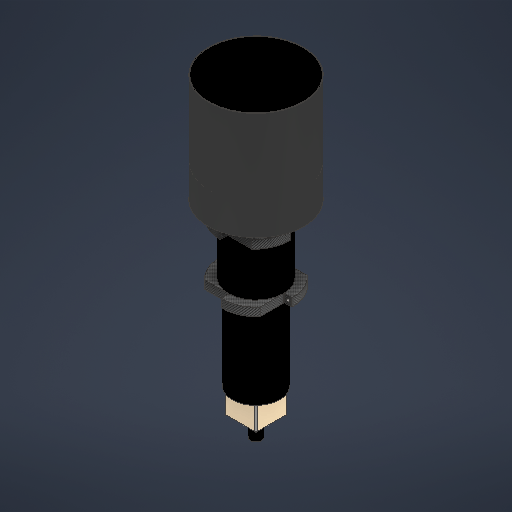
# Autodesk Inventor part: Carbon_Fibre
Saved by Autodesk Inventor 2026.2 (Build 302298000, 298)
## iProperties
Created: 2025-12-09
Part Number: Carbon_Fibre
Material: Steel
Document SubType Name: Modeling
Designer: Thoma
Density: 7.85 g/cm^3
Appearance: Semi-Polished
Mass: 18868.6 g
Surface Area: 2628.33 cm^2
Volume: 2403.64 cm^3
Author: Thoma
Autodesk Inventor part; units mm, degrees
ref_plane "YZ Plane" through (0, 0, 0) normal (1, 0, 0) x (0, 1, 0)
ref_plane "XZ Plane" through (0, 0, 0) normal (0, 1, 0) x (-1, 0, 0)
ref_plane "XY Plane" through (0, 0, 0) normal (0, 0, 1) x (1, 0, 0)
sketch "Sketch1" plane through (0, 0, 0) normal (0, 1, 0) x (-1, 0, 0)
  circle A0 centre (0, 0) radius 43.5
  dimension "d0" = 87
  constraints: 1 centre point, 1 coincident
  measures "d0" diameter of A0
extrude "Extrusion1" add sketch "Sketch1" along normal blind 13
sketch "Sketch2" plane through (0, 13, 0) normal (0, 1, 0) x (1, 0, 0)
  circle A0 centre (0, 0) radius 43.5 projected
  line L0 (0, 55.4914) -> (0, 55.5)
  circle A1 centre (0, 0) radius 43.5 projected
  line L1 (43.5, 0) -> (43.5, 37)
  line L2 (0, 55.5) -> (1, 55.5)
  line L3 (1, 55.5) -> (1, 43.5)
  line L4 (0, 55.4914) -> (0, 55.5)
  arc A2 (43.5, 37) -> (1, 55.5) centre (1, -2.5676) ccw
  line L5 (1, 43.4885) -> (1, 43.5)
  line L6 (-55.5, 1) -> (-43.5, 1)
  arc A3 (-37, 43.5) -> (-55.5, 1) centre (2.5676, 1) ccw
  line L7 (0, 43.5) -> (-37, 43.5)
  line L8 (-1, -55.5) -> (-1, -43.5)
  arc A4 (-43.5, -37) -> (-1, -55.5) centre (-1, 2.5676) ccw
  line L9 (-43.5, 0) -> (-43.5, -37)
  line L10 (55.5, -1) -> (43.5, -1)
  arc A5 (37, -43.5) -> (55.5, -1) centre (-2.5676, -1) ccw
  line L11 (0, -43.5) -> (37, -43.5)
  point P0 (0, 43.5)
  point P1 (43.5, 0)
  point P2 (-55.4914, 0)
  point P3 (0, -55.4914)
  point P4 (55.4914, 0)
  dimension "d3" = 12
  dimension "d75" = 1
  dimension "d91" = 37
  dimension "d92" = 58.0676
  dimension "d93" = 42.5
  dimension "d94" = 0
  dimension "d95" = 87.5
  dimension "d110" = 360
  constraints: 24 end point, 13 point on circle, 4 centre point, 4 vertical, 1 horizontal, 1 parallel, 1 perpendicular, 1 tangent, 39 other
  measures "d3" distance of A1.start L0.end
  measures "d75" distance of L0.end L2.end
  measures "d91" distance of L1.start L1.end
  measures "d92" radius of A2
  measures "d93" distance between parallel lines of L3 L1
  measures "d94" distance from line of point (43.5, 0) L1
extrude "Extrusion2" add sketch "Sketch2" against normal blind 13 contours A0 L5 L3 A2 L1
sketch "Sketch6" plane through (0, 0, 0) normal (0, -1, 0) x (1, 0, 0)
  circle A0 centre (0, 0) radius 43.5
  point P0 (0, 43.5)
  constraints: 1 coincident, 1 vertical alignment, 2 other
sketch "Sketch17" plane through (0, 13, 0) normal (0, 1, 0) x (1, 0, 0)
  circle A0 centre (0, 0) radius 25
  dimension "d141" = 50
  constraints: 1 centre point, 1 coincident
  measures "d141" diameter of A0
extrude "Extrusion16" add sketch "Sketch17" along normal blind 2
sketch "Sketch7" plane through (0, 13, 0) normal (0, 1, 0) x (1, 0, 0)
  circle A0 centre (0, 0) radius 37.5
  dimension "d23" = 75
  constraints: 1 centre point, 1 coincident
  measures "d23" diameter of A0
extrude "Extrusion5" add sketch "Sketch7" along normal blind 15
extrude "Extrusion6" add sketch "Sketch6" along normal blind 79
sketch "Sketch8" plane through (0, -79, 0) normal (0, -1, 0) x (1, 0, 0)
  line L0 (0, -43.5) -> (0, -55.5) projected
  line L1 (0, -43.4937) -> (0, -55.5)
  line L2 (43.4937, 0) -> (55.5, 0)
  line L3 (0, 43.4937) -> (0, 55.5)
  line L4 (-43.4937, 0) -> (-55.5, 0)
  line L5 (-55.5, -2) -> (-43.5, -2)
  circle A0 centre (0, 0) radius 43.5
  line L6 (-43.5, 0) -> (-55.5, 0) projected
  line L7 (-55.5, 0) -> (-55.5, -2)
  line L8 (-43.5, 0) -> (-43.5, -37)
  circle A1 centre (0, 0) radius 43.5 projected
  line L9 (-55.5, 0) -> (-55.5, 1)
  line L10 (-55.5, 1) -> (-43.4885, 1)
  line L11 (0, -43.5) -> (37, -43.5)
  line L12 (-1, -55.5) -> (-1, -43.4885)
  line L13 (2, -55.5) -> (2, -43.5)
  line L14 (0, -55.5) -> (2, -55.5)
  line L15 (0, -55.5) -> (-1, -55.5)
  circle A2 centre (0, 0) radius 43.5
  line L16 (43.5, 0) -> (43.5, 37)
  line L17 (55.5, -1) -> (43.4885, -1)
  line L18 (55.5, 2) -> (43.5, 2)
  line L19 (55.5, 0) -> (55.5, 2)
  line L20 (55.5, 0) -> (55.5, -1)
  circle A3 centre (0, 0) radius 43.5
  line L21 (0, 43.5) -> (-37, 43.5)
  line L22 (1, 55.5) -> (1, 43.4885)
  line L23 (-2, 55.5) -> (-2, 43.5)
  line L24 (0, 55.5) -> (-2, 55.5)
  line L25 (0, 55.5) -> (1, 55.5)
  circle A4 centre (0, 0) radius 43.5
  line L26 (-2, -43.5) -> (-37, -43.5) projected
  arc A5 (-43.5, -37) -> (-1, -55.5) centre (-3.75, -3.75) ccw
  arc A6 (37, -43.5) -> (55.5, -1) centre (3.75, -3.75) ccw
  line L27 (0, -43.5) -> (37, -43.5)
  line L28 (2, -55.5) -> (2, -43.5)
  line L29 (-1, -55.5) -> (-1, -43.4885)
  line L30 (0, -55.5) -> (2, -55.5)
  arc A7 (43.5, 37) -> (1, 55.5) centre (3.75, 3.75) ccw
  line L31 (43.5, 0) -> (43.5, 37)
  line L32 (55.5, 2) -> (43.5, 2)
  line L33 (55.5, -1) -> (43.4885, -1)
  line L34 (55.5, 0) -> (55.5, 2)
  arc A8 (-37, 43.5) -> (-55.5, 1) centre (-3.75, 3.75) ccw
  line L35 (0, 43.5) -> (-37, 43.5)
  line L36 (-2, 55.5) -> (-2, 43.5)
  line L37 (1, 55.5) -> (1, 43.4885)
  line L38 (0, 55.5) -> (-2, 55.5)
  line L39 (-43.5, -37) -> (0, -37)
  line L40 (0, -37) -> (0, -55.5)
  point P0 (43.5, 0)
  point P1 (0, 43.5)
  point P2 (-43.5, 0)
  point P3 (43.5, -37)
  point P4 (37, 43.5)
  point P5 (-43.5, 37)
  point P6 (43.5, 0)
  point P7 (0, 43.5)
  point P8 (-43.5, 0)
  dimension "d30" = 360
  dimension "d32" = 2
  dimension "d33" = 12
  dimension "d52" = 35
  dimension "d60" = 1
  dimension "d67" = 360
  dimension "d71" = 360
  dimension "d137" = 51.823
  dimension "d138" = 3.75
  dimension "d139" = 43.5
  dimension "d140" = 18.5
  constraints: 76 end point, 12 point on circle, 8 point on line, 4 centre point, 2 horizontal, 2 horizontal alignment, 2 perpendicular, 2 vertical, 1 coincident, 1 collinear, 1 parallel, 1 vertical alignment, 146 other
  measures "d32" distance between parallel lines of L5 L4
  measures "d33" distance of L7.start L6.start
  measures "d52" distance of L8.end L5.end
  measures "d60" distance of L7.start L9.end
  measures "d137" radius of A5
  measures "d138" horizontal distance of A5.centre point (0, 0)
  measures "d139" distance of L8.end L39.end
  measures "d140" distance of L39.end L30.start
extrude "Extrusion7" add sketch "Sketch8" along normal blind 13 contours A0 L39 L40 L1 | L1 L40 L39 A0 | A0 L17 A6 L11 | L12 A5 L39 A0 | L39 L8 A0 | A0 L22 A7 L16 | L10 A8 L21 A0
sketch "Sketch9" plane through (0, -92, 0) normal (0, -1, 0) x (1, 0, 0)
  circle A0 centre (0, 0) radius 37.5
  constraints: 1 centre point, 1 coincident
extrude "Extrusion8" add sketch "Sketch9" along normal blind 135
sketch "Sketch10" plane through (0, -227, 0) normal (0, -1, 0) x (1, 0, 0)
  line L0 (-25, 25) -> (25, 25)
  line L1 (25, 25) -> (25, -25)
  line L2 (25, -25) -> (-25, -25)
  line L3 (-25, -25) -> (-25, 25)
  point P0 (0, 0)
  point P1 (0, -25)
  dimension "d43" = 25
  dimension "d44" = 50
  dimension "d45" = 50
  dimension "d46" = 25
  constraints: 8 end point, 2 parallel, 1 horizontal, 1 midpoint, 1 perpendicular
  measures "d43" distance from line of L1 point (0, 0)
  measures "d44" distance of L0.start L0.end
  measures "d45" distance of L2.end L0.start
  measures "d46" distance of point (0, -25) point (0, 0)
extrude "Extrusion9" add sketch "Sketch10" along normal blind 40
sketch "Sketch11" plane through (0, -267, 0) normal (0, -1, 0) x (1, 0, 0)
  circle A0 centre (0, 0) radius 9
  dimension "d49" = 18
  constraints: 1 centre point, 1 coincident
  measures "d49" diameter of A0
extrude "Extrusion10" add sketch "Sketch11" along normal blind 30
pattern_circular "Circular Pattern1" count 4 over 360 about axis through (0, -10, 0) along (0, 1, 0) of "Extrusion2"
sketch "Sketch13" plane through (1, 13, -55.5) normal (-1, 0, 0) x (0, 0, 1)
  line L0 (0, 0) -> (0, -13) projected
  line L1 (0, -6.5) -> (12, -6.5)
  line L2 (12, -13) -> (12, 0) projected
  circle A0 centre (6, -6.5) radius 2.5
  point P0 (55.5, -13)
  constraints: 3 midpoint, 2 end point, 1 centre point
extrude "Extrusion12" cut sketch "Sketch13" against normal blind 10
pattern_circular "Circular Pattern2" count 4 over 360 about axis through (0, -10, 0) along (0, 1, 0) of "Extrusion12"
sketch "Sketch14" plane through (43.4885, -79, -1) normal (0, 0, 1) x (1, 0, 0)
  line L0 (12.0115, -13) -> (0, -13) projected
  line L1 (12.0115, 0) -> (0, 0) projected
  circle A0 centre (6.0115, -6.5) radius 2.5
  line L2 (0.0115, 0) -> (0.0115, -13) projected
  point P0 (-43.4885, 79)
  point P1 (6.0057, -13)
  point P2 (0.0115, -6.5)
  dimension "d120" = 5
  dimension "d128" = 6.5
  dimension "d129" = 6
  constraints: 2 midpoint, 1 centre point
  measures "d120" diameter of A0
  measures "d128" distance from line of L0 A0.centre
  measures "d129" distance from line of L2 A0.centre
extrude "Extrusion13" cut sketch "Sketch14" against normal blind 10
pattern_circular "Circular Pattern3" count 4 over 360 about axis through (0, -10, 0) along (0, 1, 0) of "Extrusion13"
fillet "Fillet1" radius 2 12 edges at (25, -227, 0) (25, -247, 25) (25, -267, 0) (25, -247, -25) (0, -267, -25) (0, -267, 25) (-25, -267, 0) (0, -227, -25) (-25, -247, -25) (-25, -227, 0) (-25, -247, 25) (0, -227, 25)
sketch "Sketch15" plane through (0, 28, 0) normal (0, 1, 0) x (1, 0, 0)
  circle A0 centre (0, 0) radius 75
  dimension "d131" = 150
  constraints: 1 centre point, 1 coincident
  measures "d131" diameter of A0
extrude "Extrusion14" add sketch "Sketch15" along normal blind 170
sketch "Sketch16" plane through (0, 198, 0) normal (0, 1, 0) x (1, 0, 0)
  circle A0 centre (0, 0) radius 9 projected
  circle A1 centre (0, 0) radius 74
  dimension "d134" = 148
  constraints: 1 centre point, 1 coincident
  measures "d134" diameter of A1
extrude "Extrusion15" cut sketch "Sketch16" against normal blind 120 contours A0 | A1
body "Solid1"
